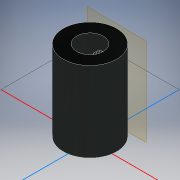
# Autodesk Inventor part: 000.002.003 - Металическая вставка
Saved by Autodesk Inventor 2022 (Build 260153000, 153)
## iProperties
Created: 2022-11-12
Part Number: 000.002.003 - Металическая вставка
Material: Сталь
Document SubType Name: Modeling
Designer: Petrov Ivan
Density: 7.85 g/cm^3
Appearance: Оружейный металл — полированный
Author: Petrov Ivan
Autodesk Inventor part; units mm, degrees
ref_plane "YZ Plane" through (0, 0, 0) normal (1, 0, 0) x (0, 1, 0)
ref_plane "XZ Plane" through (0, 0, 0) normal (0, 1, 0) x (-1, 0, 0)
sketch "Эскиз1" plane through (0, 0, 0) normal (0, 1, 0) x (-1, 0, 0)
  circle A0 centre (0, 0) radius 6
  circle A1 centre (0, 0) radius 3
  dimension "d0" = 12
  dimension "d1" = 6
  constraints: 2 centre point, 2 coincident
  measures "d0" diameter of A0
  measures "d1" diameter of A1
extrude "Выдавливание1" add sketch "Эскиз1" along normal blind 18
ref_plane "РабПлоскость1" through (0, 0, -6) normal (0, 0, 1) x (1, 0, 0)
sketch "Эскиз2" plane through (0, 0, -6) normal (0, 0, 1) x (1, 0, 0)
  circle A0 centre (0, 5) radius 2
  circle A1 centre (0, 13) radius 2
  line L0 (-6, 0) -> (-6, 18) projected
  line L1 (-6, 9) -> (-4.8427, 9) construction
  point P0 (0, 0)
  dimension "d4" = 4
  dimension "d5" = 4
  dimension "d6" = 8
  constraints: 2 centre point, 2 end point, 1 horizontal, 1 midpoint, 1 symmetric about line
  measures "d4" diameter of A0
  measures "d5" diameter of A1
  measures "d6" distance of A1.centre A0.centre
extrude "Выдавливание2" cut sketch "Эскиз2" along normal blind 4 contours A1
thread "Резьба2" size "M4x0.7" class "6H" standard "ANSI Metric M Profile" length 51.6
equation "\"d7\" = d4"
